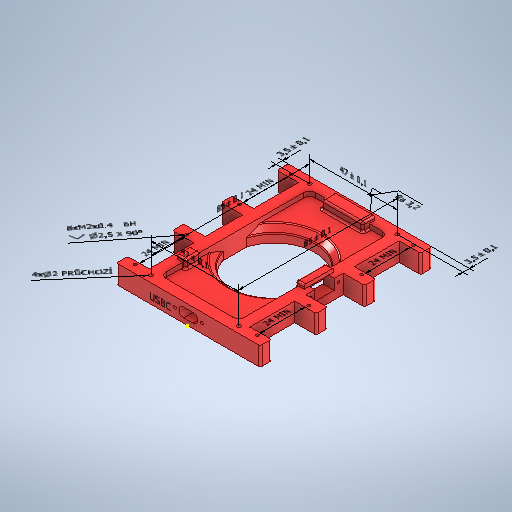
# Autodesk Inventor part: rapoukBasev5
Saved by Autodesk Inventor 2025.1 (Build 291241000, 241)
## iProperties
Created: 2024-01-02
Part Number: rapoukBasev5
Material: EN AW-6060 T6
Document SubType Name: Modeling
Designer: Roman Suk
Density: 2.7 g/cm^3
Appearance: Light Red
MASSSFP: 400 g
SFP: 4HR
Author: Roman Suk
Autodesk Inventor part; units mm, degrees
ref_plane "YZ Plane" through (0, 0, 0) normal (1, 0, 0) x (0, 1, 0)
ref_plane "XZ Plane" through (0, 0, 0) normal (0, 1, 0) x (-1, 0, 0)
sketch "Sketch2" plane through (0, 0, 0) normal (0, 1, 0) x (-1, 0, 0)
  line L0 (0, 0) -> (0, 40)
  line L1 (0, 40) -> (17.825, 40)
  line L2 (0, 40) -> (0, 46) construction
  line L3 (0, 46) -> (37.5, 46)
  line L4 (21, 36.825) -> (21, 0)
  line L5 (38.5, 45) -> (38.5, 41)
  line L6 (37.5, 40) -> (27, 40)
  line L7 (27, 40) -> (27, 16)
  line L8 (27, 16) -> (37.5, 16)
  line L9 (38.5, 15) -> (38.5, 11)
  line L10 (37.5, 10) -> (27, 10)
  line L11 (27, 10) -> (27, 0)
  line L12 (0, 0) -> (21, 0)
  line L13 (27, 28) -> (38.5, 28)
  arc A0 (21, 36.825) -> (17.825, 40) centre (17.825, 36.825) ccw
  arc A1 (38.5, 45) -> (37.5, 46) centre (37.5, 45) ccw
  arc A2 (37.5, 40) -> (38.5, 41) centre (37.5, 41) ccw
  arc A3 (38.5, 15) -> (37.5, 16) centre (37.5, 15) ccw
  arc A4 (37.5, 10) -> (38.5, 11) centre (37.5, 11) ccw
  line L14 (0, -40) -> (17.825, -40)
  line L15 (0, -46) -> (37.5, -46)
  line L16 (21, -36.825) -> (21, 0)
  line L17 (38.5, -45) -> (38.5, -41)
  line L18 (37.5, -40) -> (27, -40)
  line L19 (27, -40) -> (27, -16)
  line L20 (27, -16) -> (37.5, -16)
  line L21 (38.5, -15) -> (38.5, -11)
  line L22 (37.5, -10) -> (27, -10)
  line L23 (27, -10) -> (27, 0)
  arc A5 (17.825, -40) -> (21, -36.825) centre (17.825, -36.825) ccw
  arc A6 (37.5, -46) -> (38.5, -45) centre (37.5, -45) ccw
  arc A7 (38.5, -41) -> (37.5, -40) centre (37.5, -41) ccw
  arc A8 (37.5, -16) -> (38.5, -15) centre (37.5, -15) ccw
  arc A9 (38.5, -11) -> (37.5, -10) centre (37.5, -11) ccw
  line L24 (0, 40) -> (-17.825, 40)
  line L25 (0, 46) -> (-37.5, 46)
  line L26 (-21, 36.825) -> (-21, 0)
  line L27 (-38.5, 45) -> (-38.5, 41)
  line L28 (-37.5, 40) -> (-27, 40)
  line L29 (-27, 40) -> (-27, 16)
  line L30 (-27, 16) -> (-37.5, 16)
  line L31 (-38.5, 15) -> (-38.5, 11)
  line L32 (-37.5, 10) -> (-27, 10)
  line L33 (-27, 10) -> (-27, 0)
  arc A10 (-17.825, 40) -> (-21, 36.825) centre (-17.825, 36.825) ccw
  arc A11 (-37.5, 46) -> (-38.5, 45) centre (-37.5, 45) ccw
  arc A12 (-38.5, 41) -> (-37.5, 40) centre (-37.5, 41) ccw
  arc A13 (-37.5, 16) -> (-38.5, 15) centre (-37.5, 15) ccw
  arc A14 (-38.5, 11) -> (-37.5, 10) centre (-37.5, 11) ccw
  line L34 (0, -46) -> (-37.5, -46)
  arc A15 (-38.5, -45) -> (-37.5, -46) centre (-37.5, -45) ccw
  line L35 (-38.5, -45) -> (-38.5, -41)
  arc A16 (-37.5, -40) -> (-38.5, -41) centre (-37.5, -41) ccw
  line L36 (-37.5, -40) -> (-27, -40)
  line L37 (-27, -40) -> (-27, -16)
  line L38 (-27, -16) -> (-37.5, -16)
  arc A17 (-38.5, -15) -> (-37.5, -16) centre (-37.5, -15) ccw
  line L39 (-38.5, -15) -> (-38.5, -11)
  arc A18 (-37.5, -10) -> (-38.5, -11) centre (-37.5, -11) ccw
  line L40 (-37.5, -10) -> (-27, -10)
  line L41 (-27, -10) -> (-27, 0)
  line L42 (-21, -36.825) -> (-21, 0)
  line L43 (0, -40) -> (-17.825, -40)
  arc A19 (-21, -36.825) -> (-17.825, -40) centre (-17.825, -36.825) ccw
  line L44 (23.5, 42.5) -> (23.5, -46) construction
  point P0 (21, 40)
  point P1 (38.5, 46)
  point P2 (38.5, 40)
  point P3 (38.5, 16)
  point P4 (38.5, 10)
  point P5 (32.74, 41.8)
  point P6 (32.74, 14.2)
  point P7 (32.74, -41.8)
  point P8 (32.74, -14.2)
  point P9 (-32.74, 41.8)
  point P10 (-32.74, 14.2)
  point P11 (-32.74, -41.8)
  point P12 (-32.74, -14.2)
  point P13 (-23.5, 42.5)
  point P14 (23.5, -42.5)
  point P15 (-23.5, 42.5)
  point P16 (-23.5, -42.5)
  dimension "d2" = 40
  dimension "d3" = 6
  dimension "d4" = 38.5
  dimension "d5" = 21
  dimension "d6" = 6
  dimension "d7" = 11.5
  dimension "d8" = 24
  dimension "d9" = 11.5
  dimension "d10" = 6
  dimension "d11" = 11.5
  dimension "d12" = 5.74
  dimension "d13" = 27.6
  dimension "d14" = 3.175
  dimension "d15" = 1
  dimension "d37" = 47
  dimension "d174" = 85
  dimension "d176" = 92
  dimension "d177" = 3.5
  constraints: 90 end point, 68 symmetric about line, 40 point on circle, 20 centre point, 16 point on line, 10 tangent, 5 perpendicular, 5 vertical, 4 horizontal, 3 equal radius, 1 midpoint, 15 other
  measures "d2" distance of L0.start L0.end
  measures "d3" distance of L0.end L2.end
  measures "d4" distance of L2.end point (38.5, 46)
  measures "d5" distance of L0.end point (21, 40)
  measures "d6" distance of point (38.5, 46) point (38.5, 40)
  measures "d7" distance of point (38.5, 40) L6.end
  measures "d8" distance of L6.end L7.end
  measures "d9" distance of L7.end point (38.5, 16)
  measures "d10" distance of point (38.5, 16) point (38.5, 10)
  measures "d11" distance of point (38.5, 10) L10.end
  measures "d12" distance from line of point (32.74, 41.8) L7
  measures "d13" diameter of point (32.74, 41.8) L13
  measures "d14" radius of A0
  measures "d15" radius of A1
  measures "d37" diameter of L44.start L0
  measures "d174" distance of L44.start point (23.5, -42.5)
  measures "d176" distance between parallel lines of L25 L34
  measures "d177" distance from line of L15 point (23.5, -42.5)
extrude "Extrusion2" add sketch "Sketch2" along normal blind 10
hole "Hole1" at (-32.74, 0, 41.8) at (-32.74, 0, 14.2) at (-32.74, 0, -41.8) at (-32.74, 0, -14.2) at (32.74, 0, 41.8) at (32.74, 0, 14.2) at (32.74, 0, -14.2) at (32.74, 0, -41.8) direction (0, 1, 0) diameter 1.567 end through all countersink diameter 2.5 countersink angle 90 thread size "M2x0.4" class "6H" standard "ISO Metric profile"
hole "Hole2" at (-23.5, 0, 42.5) at (23.5, 0, 42.5) at (-23.5, 0, -42.5) at (23.5, 0, -42.5) direction (0, 1, 0) diameter 2 end through all
sketch "Sketch4" plane through (-37.5, 0, 46) normal (0, 0, 1) x (1, 0, 0)
  line L0 (37.5, 0) -> (37.5, 10) construction
  line L1 (0, 10) -> (75, 10) projected
  line L2 (-1, 0) -> (-1, 10) projected
  line L3 (-1, 5) -> (75, 5)
  line L4 (35, 5) -> (40, 5) construction
  line L5 (35, 2.5) -> (40, 2.5)
  line L6 (40, 7.5) -> (35, 7.5)
  arc A0 (35, 7.5) -> (35, 2.5) centre (35, 5) ccw
  arc A1 (40, 2.5) -> (40, 7.5) centre (40, 5) ccw
  point P0 (37.5, 5)
  point P1 (42.5, 5)
  point P2 (32.5, 5)
  point P3 (30.25, 5)
  point P4 (44.75, 5)
  dimension "d189" = 2.5
  dimension "d190" = 5
  dimension "d191" = 10
  dimension "d192" = 14.5
  constraints: 12 end point, 6 point on circle, 4 midpoint, 4 tangent, 2 centre point, 2 point on line, 1 horizontal, 1 parallel, 1 symmetric about line
  measures "d189" distance of point (37.5, 5) L4.end
  measures "d190" diameter of A1
  measures "d191" distance of point (42.5, 5) point (32.5, 5)
  measures "d192" diameter of point (30.25, 5) L0
extrude "Extrusion3" cut sketch "Sketch4" against normal up to surface (6 mm away)
sketch "Sketch6" plane through (37.5, 0, -46) normal (0, 0, -1) x (-1, 0, 0)
  line L0 (0, 0) -> (0, 10) projected
  line L1 (0, 5) -> (75, 5)
  line L2 (75, 0) -> (75, 10) projected
  line L3 (37.5, 0) -> (37.5, 10) construction
  line L4 (31.4, 2.2) -> (43.6, 2.2)
  line L5 (44.6, 3.2) -> (44.6, 6.8)
  line L6 (43.6, 7.8) -> (31.4, 7.8)
  line L7 (30.4, 6.8) -> (30.4, 3.2)
  line L8 (30.4, 2.2) -> (44.6, 7.8) construction
  line L9 (44.6, 2.2) -> (30.4, 7.8) construction
  line L10 (0, 10) -> (75, 10) projected
  line L11 (75, 0) -> (75, 10) projected
  arc A0 (43.6, 2.2) -> (44.6, 3.2) centre (43.6, 3.2) ccw
  arc A1 (30.4, 3.2) -> (31.4, 2.2) centre (31.4, 3.2) ccw
  arc A2 (31.4, 7.8) -> (30.4, 6.8) centre (31.4, 6.8) ccw
  arc A3 (44.6, 6.8) -> (43.6, 7.8) centre (43.6, 6.8) ccw
  line L12 (33.95, 7.8) -> (33.95, 2.2) construction
  line L13 (41.05, 7.8) -> (41.05, 2.2) construction
  circle A4 centre (33.95, 5) radius 2.8
  circle A5 centre (41.05, 5) radius 2.8
  point P0 (37.5, 5)
  point P1 (37.5, 5)
  point P2 (41.05, 2.2)
  point P3 (33.95, 2.2)
  dimension "d169" = 14.2
  dimension "d170" = 5.6
  dimension "d173" = 1
  dimension "d186" = 7.1
  constraints: 20 end point, 10 midpoint, 10 point on line, 8 point on circle, 8 tangent, 4 centre point, 3 equal radius, 2 parallel, 2 perpendicular, 2 symmetric about line, 1 horizontal, 1 horizontal alignment, 1 vertical, 1 vertical alignment, 6 other
  measures "d169" distance of L9.end L8.end
  measures "d170" distance of L8.end L9.start
  measures "d173" radius of A0
  measures "d186" diameter of point (37.5, 5) L12
extrude "Extrusion4" cut sketch "Sketch6" against normal up to surface (6 mm away) contours A4 L1 | L1 A4 | A5 L1 | L1 A5
extrude "Vysunutí5" cut sketch "Sketch6" against normal blind 5 contours L7 A2 L6 A4 L1 | L1 A4 L4 A1 L7 | A4 L6 A5 L1 | L1 A5 L4 A4 | L5 A0 L4 A5 L1 | L1 A5 L6 A3 L5
hole "Díra4" at (-7.25, 5, 46) at (7.25, 5, 46) direction (0, 0, -1) diameter 1.567 depth 6 thread size "M2x0.4" class "6H" standard "ISO Metric profile"
sketch "Náčrt7" plane through (27, 0, 10) normal (1, 0, 0) x (0, 0, -1)
  line L0 (10, 0) -> (10, 10) construction
  line L1 (0, 10) -> (20, 10) projected
  line L2 (15.25, 4.4) -> (4.75, 4.4)
  line L3 (4.75, 4.4) -> (4.75, 10)
  line L4 (4.75, 10) -> (15.25, 10)
  line L5 (15.25, 10) -> (15.25, 4.4)
  line L6 (15.25, 4.4) -> (4.75, 10) construction
  line L7 (4.75, 4.4) -> (15.25, 10) construction
  point P0 (10, 7.2)
  point P1 (2.5, 7.2)
  point P2 (17.5, 7.2)
  dimension "d200" = 5.6
  dimension "d201" = 10.5
  dimension "d202" = 15
  constraints: 14 end point, 3 midpoint, 2 parallel, 2 point on line, 1 horizontal, 1 horizontal alignment, 1 perpendicular, 1 symmetric about line
  measures "d200" distance between parallel lines of L1 L2
  measures "d201" distance between parallel lines of L5 L3
  measures "d202" diameter of point (2.5, 7.2) L0
hole "Díra5" at (27, 7.2, 7.5) at (27, 7.2, -7.5) direction (-1, 0, 0) diameter 1.567 depth 6 thread size "M2x0.4" class "6H" standard "ISO Metric profile"
extrude "Vysunutí6" cut sketch "Náčrt7" against normal up to surface (6 mm away)
sketch "Náčrt8" plane through (-37.5, 0, 46) normal (0, 0, 1) x (1, 0, 0)
  circle A0 centre (30.25, 5) radius 0.7835 projected
  line L0 (29.4665, 5) -> (29.4665, 10)
  line L1 (0, 10) -> (75, 10) projected
  circle A1 centre (44.75, 5) radius 0.7835 projected
  line L2 (45.5335, 5) -> (45.5335, 10)
  circle A2 centre (30.25, 5) radius 1
  circle A3 centre (44.75, 5) radius 1
  line L3 (29.25, 5) -> (29.25, 10)
  line L4 (45.75, 5) -> (45.75, 10)
  point P0 (37.5, 0)
  dimension "d213" = 2
  dimension "d214" = 2
  dimension "d212" = 16.067
  dimension "d215" = 16.5
  constraints: 8 end point, 5 vertical, 4 horizontal alignment, 4 point on line, 3 perpendicular, 2 coincident, 6 other
  measures "d212" distance between parallel lines of L2 L0
  measures "d215" distance between parallel lines of L4 L3
sketch "Náčrt9" plane through (0, 0, 0) normal (0, -1, 0) x (1, 0, 0)
  line L0 (18, -40) -> (-18, -40)
  line L1 (-21, -37) -> (-21, 37)
  line L2 (-18, 40) -> (18, 40)
  line L3 (21, 37) -> (21, -37)
  line L4 (21, -40) -> (-21, 40) construction
  line L5 (-21, -40) -> (21, 40) construction
  arc A0 (-21, -37) -> (-18, -40) centre (-18, -37) ccw
  arc A1 (18, -40) -> (21, -37) centre (18, -37) ccw
  arc A2 (21, 37) -> (18, 40) centre (18, 37) ccw
  arc A3 (-18, 40) -> (-21, 37) centre (-18, 37) ccw
  circle A4 centre (0, 0) radius 21.9
  circle A5 centre (0, 0) radius 10
  line L6 (11, -40) -> (-11, -40)
  line L7 (-11, -40) -> (-11, -36.5)
  line L8 (-11, -36.5) -> (11, -36.5)
  line L9 (11, -36.5) -> (11, -40)
  line L10 (11, -40) -> (-11, -36.5) construction
  line L11 (-11, -40) -> (11, -36.5) construction
  point P0 (-21, 36.825)
  point P1 (-17.825, 40)
  point P2 (0, -38.25)
  point P3 (-11, -38.25)
  point P4 (0, -40)
  point P5 (-21, 6.2137)
  point P6 (21, 6.2137)
  point P7 (-11, -40)
  point P8 (21, -6.2137)
  point P9 (-21, -6.2137)
  dimension "d216" = 3
  dimension "d217" = 43.8
  dimension "d218" = 20
  dimension "d219" = 22
  dimension "d220" = 3.5
  constraints: 24 end point, 8 point on circle, 8 point on line, 8 tangent, 6 centre point, 6 midpoint, 4 parallel, 3 equal radius, 2 coincident, 2 horizontal, 2 horizontal alignment, 2 perpendicular, 2 vertical alignment
  measures "d216" radius of A0
  measures "d217" diameter of A4
  measures "d218" diameter of A5
  measures "d219" distance from line of L9 point (-11, -38.25)
  measures "d220" distance between parallel lines of L8 L6
extrude "Vysunutí7" add sketch "Náčrt9" against normal blind 7.5 separate body contours L0 L9 L8 L7 A0 L1 A4 L3 A1 | A4 L1 A3 L2 A2 L3
extrude "Vysunutí8" add sketch "Náčrt9" against normal blind 12 separate body contours L0 L7 L8 L9
combine bodies "Kombinovat1" operation type add bodies to combine 3 2
chamfer "Zkosení1" distance 3 angle 45 2 edges at (0, 7.5, -21.9) (0, 7.5, 21.9)
sketch "Náčrt10" plane through (18, 0, -40) normal (0, 0, -1) x (-1, 0, 0)
  line L0 (7, 12) -> (29, 12) projected
  line L1 (-19.5, 10) -> (55.5, 10) projected
  line L2 (29, 12) -> (7, 12)
  line L3 (7, 12) -> (7, 10)
  line L4 (7, 10) -> (29, 10)
  line L5 (29, 10) -> (29, 12)
  point P0 (18, 0)
  constraints: 8 end point, 2 parallel, 1 coincident, 1 horizontal, 1 perpendicular, 1 point on line
extrude "Vysunutí9" add sketch "Náčrt10" along normal blind 3 separate body
combine bodies "Kombinovat2" operation type add bodies to combine 3 4
sketch "Náčrt11" plane through (-18, 7.5, 40) normal (0, 1, 0) x (1, 0, 0)
  line L0 (-3, 3.175) -> (-3, 76.825) projected
  line L1 (-3, 12) -> (-1.5, 12)
  line L2 (-1.5, 12) -> (-1.5, 20)
  line L3 (-1.5, 20) -> (-3, 20)
  line L4 (-3, 20) -> (-3, 12)
  line L5 (35.825, 0) -> (0.175, 0) projected
  point P0 (18, 40)
  point P1 (-3, 20)
  dimension "d232" = 1.5
  dimension "d233" = 8
  dimension "d234" = 12
  constraints: 8 end point, 2 parallel, 1 horizontal, 1 perpendicular, 1 point on line
  measures "d232" distance of L3.end L2.end
  measures "d233" distance of L2.end L1.end
  measures "d234" distance between parallel lines of L5 L1
extrude "Vysunutí10" add sketch "Náčrt11" along normal up to surface (4.5 mm away) separate body
sketch "Náčrt12" plane through (-21, 7.5, 20) normal (-1, 0, 0) x (0, 0, 1)
  line L0 (0, 4.5) -> (8, 4.5) projected
  line L1 (20, 2.5) -> (-4, 2.5) projected
  line L2 (8, 4.5) -> (0, 4.5)
  line L3 (0, 4.5) -> (0, 2.5)
  line L4 (0, 2.5) -> (8, 2.5)
  line L5 (8, 2.5) -> (8, 4.5)
  point P0 (-20, -7.5)
  constraints: 8 end point, 2 parallel, 1 coincident, 1 horizontal, 1 perpendicular, 1 point on line
extrude "Vysunutí11" add sketch "Náčrt12" along normal blind 3 separate body
combine bodies "Kombinovat3" operation type add bodies to combine 6 5
combine bodies "Kombinovat4" operation type add bodies to combine 6 3
ref_plane "Pracovní rovina1" through (27, 4.4, 0) normal (0, 0, -1) x (-1, 0, 0)
sketch "Náčrt13" plane through (27, 4.4, 0) normal (0, 0, -1) x (-1, 0, 0)
  line L0 (2.5, 5.6) -> (4.5, 5.6) projected
  line L1 (6, 5.6) -> (6, 0) projected
  line L2 (6, 5.6) -> (3, 5.6)
  line L3 (0, 5.6) -> (6, 5.6) projected
  line L4 (3, 5.6) -> (3, 7.6)
  line L5 (3, 7.6) -> (7.5, 7.6)
  line L6 (7.5, 7.6) -> (7.5, 4.5981)
  line L7 (7.5, 4.5981) -> (6, 2)
  line L8 (0, 0) -> (6, 0) projected
  line L9 (6, 0) -> (6, 2)
  line L10 (6, 5.6) -> (6, 4.1374)
  line L11 (6, 5.6) -> (6.4441, 5.6)
  line L12 (6.4441, 5.6) -> (6.4441, 3.6)
  line L13 (6.4441, 3.6) -> (6, 3.6)
  line L14 (6, 3.6) -> (6, 5.6)
  point P0 (27, -4.4)
  point P1 (3, 5.6)
  point P2 (6, 4.6)
  point P3 (6.2221, 5.6)
  point P4 (6.2221, 3.6)
  point P5 (6, 3.6)
  dimension "d240" = 2
  dimension "d241" = 2
  dimension "d242" = 1.5
  dimension "d243" = 30
  dimension "d246" = 0.4441
  dimension "d247" = 2
  constraints: 22 end point, 4 midpoint, 2 horizontal, 2 parallel, 2 perpendicular, 2 point on line, 1 collinear, 1 vertical
  measures "d240" distance between parallel lines of L5 L2
  measures "d241" distance from line of L8 L7.end
  measures "d242" distance between parallel lines of L1 L6
  measures "d243" angle of L1 L7
  measures "d246" distance from line of point (6, 4.6) L12
  measures "d247" distance of point (6.222, 5.6) point (6.222, 3.6)
extrude "Vysunutí12" add sketch "Náčrt13" along normal mid plane 16 separate body contours L4 L5 L6 L7 L1 L13 L12 L11 L2 L0
fillet "Zaoblení2" radius 1 28 edges at (-11, 7.5, -38.25) (0, 7.5, -36.5) (0, 12, -36.5) (-11, 9.75, -36.5) (11, 9.75, -36.5) (11, 7.5, -38.25) (-11, 12, -39.75) (11, 12, -39.75) (0, 4.5, 21.9) (0, 7.5, 24.9) (0, 7.5, -24.9) (0, 4.5, -21.9) (-19.5, 12, 24) (-21.75, 12, 28) (-21.75, 12, 20) (-19.5, 7.5, 24) (-19.5, 9.75, 20) (-20.25, 7.5, 20) (-19.5, 9.75, 28) (-20.25, 7.5, 28) (19.5, 8.9981, 0) (20.25, 7.699, -8) (19.5, 10.499, -8) (21.75, 12, -8) (19.5, 12, 0) (21.75, 12, 8) (19.5, 10.499, 8) (20.25, 7.699, 8)
sketch "Náčrt14" plane through (37.5, 0, -46) normal (0, 0, -1) x (-1, 0, 0)
  line L0 (12.7336, 6.1909) -> (35.9669, 6.1909) construction
  line L1 (35.9669, 6.1909) -> (35.9669, -2.6246) construction
  line L2 (35.9669, -2.6246) -> (12.7336, -2.6246) construction
  line L3 (12.7336, -2.6246) -> (12.7336, 6.1909) construction
  point P0 (37.5, 0)
  constraints: 2 other
sketch "Náčrt15" plane through (-37.5, 0, 46) normal (0, 0, 1) x (1, 0, 0)
  line L0 (16.5467, 5.5722) -> (40.6129, 5.5722) construction
  line L1 (40.6129, 5.5722) -> (40.6129, -2.7434) construction
  line L2 (40.6129, -2.7434) -> (16.5467, -2.7434) construction
  line L3 (16.5467, -2.7434) -> (16.5467, 5.5722) construction
  point P0 (37.5, 0)
  constraints: 2 other
equation "\"d6\" = d3"
equation "\"d9\" = d7"
equation "\"d10\" = d3"
equation "\"d11\" = d7"
body "Solid2"
